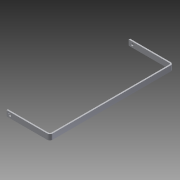
# Autodesk Inventor part: tie-together tier 2
Saved by Autodesk Inventor 2013 (Build 170138000, 138)
## iProperties
Created: 2013-01-24
Part Number: tie-together tier 2
Material: Aluminum 6061
Document SubType Name: Sheet Metal
Designer: Arpan
Density: 2.71 g/cm^3
Sheet Metal Rule: Default
Mass: 50.0858 g
Surface Area: 149.653 cm^2
Volume: 18.4818 cm^3
Author: Arpan
Autodesk Inventor part; units mm, degrees
ref_plane "YZ Plane" through (0, 0, 0) normal (1, 0, 0) x (0, 1, 0)
ref_plane "XZ Plane" through (0, 0, 0) normal (0, 1, 0) x (-1, 0, 0)
ref_plane "XY Plane" through (0, 0, 0) normal (0, 0, 1) x (1, 0, 0)
sketch "Sketch1" plane through (0, 0, 0) normal (0, 0, 1) x (1, 0, 0)
  line L0 (0, 0) -> (-95.0976, 0)
  line L1 (-95.0976, 0) -> (-95.0976, 12.7)
  line L2 (-95.0976, 12.7) -> (0, 12.7)
  line L3 (0, 12.7) -> (0, 0)
  line L4 (0, 12.7) -> (-45.593, 12.7)
  line L5 (-95.0976, 12.7) -> (-87.6046, 12.7)
  dimension "d1" = 95.0976
  dimension "d2" = 12.7
  dimension "d5" = 7.493
  constraints: 12 end point, 2 perpendicular, 2 point on line, 1 horizontal, 1 parallel
  measures "d1" distance of L0.start L0.end
  measures "d2" distance of L0.end L1.end
  measures "d5" distance of L1.end L5.end
extrude "Plate5" add sketch "Sketch1" along normal blind 3.175
sketch "Sketch6" plane through (3.175, 0, -3.175) normal (1, 0, 0) x (0, 1, 0)
  line L0 (12.7, 0) -> (0, 0)
  line L1 (0, 0) -> (0, -276.6822)
  line L2 (0, -276.6822) -> (12.7, -276.6822)
  line L3 (12.7, -276.6822) -> (12.7, 0)
  constraints: 6 end point, 1 horizontal, 1 perpendicular, 1 vertical
edge flange "Flange4" height 283.0322 angle 90 thickness 3.175 bend radius 3.175 thickness toward (1, 0, 0) relief straight relief width 3.175 relief depth 1.5875 edges at (0, 6.35, 0) wall of the first edge with corners at (3.175, 12.7, -3.175) (3.175, 0, -3.175) (3.175, 0, -279.8572) (3.175, 12.7, -279.8572)
bend "Bend4"
corner "Corner4"
sketch "Sketch7" plane through (0, 0, -283.0322) normal (0, 0, -1) x (-1, 0, 0)
  line L0 (0, 12.7) -> (0, 0)
  line L1 (0, 0) -> (95.0976, 0)
  line L2 (95.0976, 0) -> (95.0976, 12.7)
  line L3 (95.0976, 12.7) -> (0, 12.7)
  constraints: 6 end point, 1 horizontal, 1 perpendicular, 1 vertical
edge flange "Flange5" height 101.4476 angle 90 thickness 3.175 bend radius 3.175 thickness toward (0, 0, -1) relief straight relief width 3.175 relief depth 1.5875 edges at (3.175, 6.35, -279.8572) wall of the first edge with corners at (0, 12.7, -283.0322) (0, 0, -283.0322) (-95.0976, 0, -283.0322) (-95.0976, 12.7, -283.0322)
bend "Bend5"
corner "Corner5"
sketch "Sketch12" plane through (0, 0, 3.175) normal (0, 0, 1) x (1, 0, 0)
  line L0 (0, 12.7) -> (0, 0) projected
  line L1 (-95.0976, 0) -> (-95.0976, 12.7) projected
  line L2 (0, 6.35) -> (-87.6046, 6.35)
  circle A0 centre (-87.6046, 6.35) radius 3.302
  line L3 (0, 6.35) -> (-40.3301, 6.35)
  line L4 (0, 6.35) -> (-45.6122, 6.35)
  dimension "d66" = 6.604
  dimension "d67" = 7.493
  dimension "d70" = 49.4854
  constraints: 6 end point, 2 point on line, 1 centre point, 1 coincident, 1 midpoint, 1 perpendicular
  measures "d66" diameter of A0
  measures "d67" distance from line of L1 L2.end
  measures "d70" distance from line of L1 L4.end
extrude "Extrusion3" cut sketch "Sketch12" against normal blind 25374.6
sketch "Sketch13" plane through (0, 0, 3.175) normal (0, 0, 1) x (1, 0, 0)
  circle A0 centre (-45.6046, 6.35) radius 3.3 projected
  circle A1 centre (-45.6046, 6.35) radius 3.3 projected
extrude "Cut1" cut sketch "Sketch13" against normal blind 3.175
sketch "Sketch14" plane through (0, 0, 3.175) normal (0, 0, 1) x (1, 0, 0)
  circle A0 centre (-45.6046, 6.35) radius 3.3 projected
extrude "Extrusion4" cut sketch "Sketch14" against normal blind 508
equation "\"d73\" = Thickness"
equation "\"d43\" = BendReliefWidth"
equation "\"d44\" = BendReliefDepth"
equation "\"d45\" = MinimumRemnant"
equation "\"d46\" = BendRadius"
equation "\"d49\" = BendRadius"
equation "\"d50\" = CornerReliefSize"
equation "\"d51\" = GapSize"
equation "\"d52\" = JacobiRadiusSize"
equation "\"d53\" = BendReliefWidth"
equation "\"d54\" = BendReliefDepth"
equation "\"d55\" = MinimumRemnant"
equation "\"d56\" = BendRadius"
equation "\"d59\" = BendRadius"
equation "\"d60\" = CornerReliefSize"
equation "\"d61\" = GapSize"
equation "\"d62\" = JacobiRadiusSize"
equation "\"BendRadius\" = Thickness"
equation "\"BendReliefWidth\" = Thickness"
equation "\"BendReliefDepth\" = 0.5 * Thickness"
equation "\"CornerReliefSize\" = 4 * Thickness"
equation "\"MinimumRemnant\" = 2 * Thickness"
equation "\"TransitionRadius\" = BendRadius"
equation "\"JacobiRadiusSize\" = BendRadius"
equation "\"GapSize\" = Thickness"
equation "\"d8\" = BendRadius"
equation "\"d42\" = BendRadius"
equation "\"Thickness\" = 3.175"
body "Solid2"
